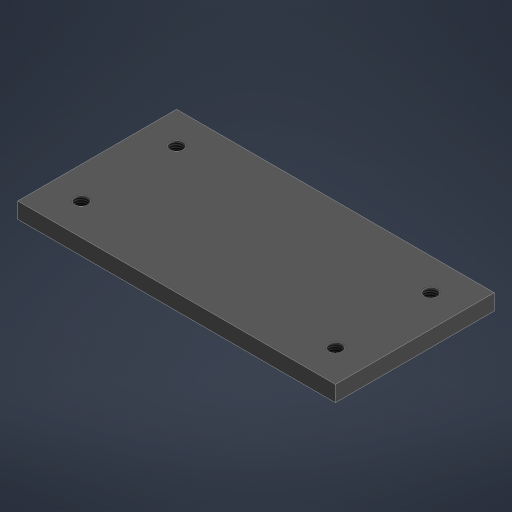
# Autodesk Inventor part: Groundplate
Saved by Autodesk Inventor 2023 (Build 270158000, 158)
## iProperties
Created: 2021-12-04
Part Number: Groundplate
Material: Generic
Document SubType Name: Modeling
Designer: LEGION SMIT
Density: 1 g/cm^3
Appearance: Generic
Author: LEGION SMIT
Autodesk Inventor part; units mm, degrees
ref_plane "YZ Plane" through (0, 0, 0) normal (1, 0, 0) x (0, 1, 0)
ref_plane "XZ Plane" through (0, 0, 0) normal (0, 1, 0) x (-1, 0, 0)
ref_plane "XY Plane" through (0, 0, 0) normal (0, 0, 1) x (1, 0, 0)
sketch "Sketch1" plane through (0, 0, 0) normal (0, 1, 0) x (-1, 0, 0)
  line L0 (50, -25) -> (-50, -25)
  line L1 (-50, -25) -> (-50, 25)
  line L2 (-50, 25) -> (50, 25)
  line L3 (50, 25) -> (50, -25)
  line L4 (50, -25) -> (-50, 25) construction
  line L5 (-50, -25) -> (50, 25) construction
  point P0 (0, 0)
  dimension "d0" = 100
  dimension "d1" = 50
  constraints: 12 end point, 2 midpoint, 2 parallel, 1 horizontal, 1 perpendicular
  measures "d0" distance of L1.end L2.end
  measures "d1" distance of L0.end L1.end
extrude "Extrusion1" add sketch "Sketch1" along normal blind 5
sketch "Sketch3" plane through (0, 5, 0) normal (0, 1, 0) x (1, 0, 0)
  line L0 (-40, 15) -> (40, 15) construction
  line L1 (40, 15) -> (40, -15) construction
  line L2 (40, -15) -> (-40, -15) construction
  line L3 (-40, -15) -> (-40, 15) construction
  line L4 (-40, 15) -> (40, -15) construction
  line L5 (40, 15) -> (-40, -15) construction
  point P0 (0, 0)
  dimension "d13" = 80
  dimension "d14" = 30
  constraints: 12 end point, 2 midpoint, 2 parallel, 1 horizontal, 1 perpendicular
  measures "d13" distance of L1.end L2.end
  measures "d14" distance of L0.end L1.end
hole "Hole2" at (-40, 5, -15) at (-40, 5, 15) at (40, 5, 15) at (40, 5, -15) direction (0, -1, 0) diameter 4 depth 6
thread "Thread1" size "M4x0.7" class "6H" standard "ANSI Metric M Profile" length 5
thread "Thread2" size "M4x0.7" class "6H" standard "ANSI Metric M Profile" length 5
thread "Thread3" size "M4x0.7" class "6H" standard "ANSI Metric M Profile" length 5
thread "Thread4" size "M4x0.7" class "6H" standard "ANSI Metric M Profile" length 5
body "Solid1"
